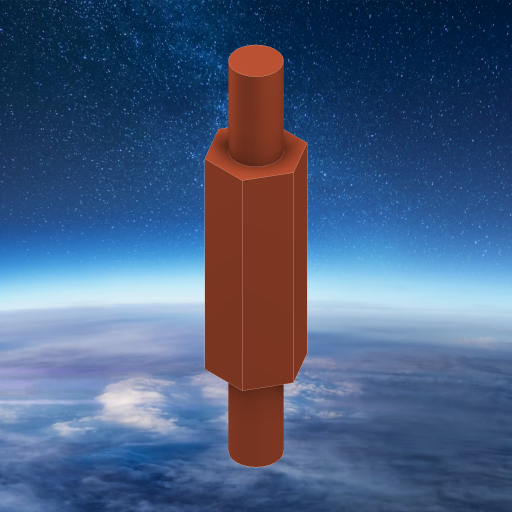
# Autodesk Inventor part: copper_pillar_M3_L15
Saved by Autodesk Inventor 2023 (Build 270158000, 158)
## iProperties
Created: 2022-11-08
Part Number: copper_pillar_M3_L15
Material: Copper
Document SubType Name: Modeling
Designer: 310611102
Density: 8.94 g/cm^3
Appearance: Copper - Satin
Mass: 3.46811 g
Surface Area: 3.98886 cm^2
Volume: 0.387932 cm^3
Author: 310611102
Autodesk Inventor part; units mm, degrees
ref_plane "YZ Plane" through (0, 0, 0) normal (1, 0, 0) x (0, 1, 0)
ref_plane "XZ Plane" through (0, 0, 0) normal (0, 1, 0) x (-1, 0, 0)
ref_plane "XY Plane" through (0, 0, 0) normal (0, 0, 1) x (1, 0, 0)
sketch "草圖2" plane through (0, 0, 0) normal (0, 1, 0) x (-1, 0, 0)
  line L0 (-2.8868, 0) -> (-1.4434, 2.5)
  line L1 (-1.4434, 2.5) -> (1.4434, 2.5)
  line L2 (1.4434, 2.5) -> (2.8868, 0)
  line L3 (2.8868, 0) -> (1.4434, -2.5)
  line L4 (1.4434, -2.5) -> (-1.4434, -2.5)
  line L5 (-1.4434, -2.5) -> (-2.8868, 0)
  point P0 (0, 0)
  point P1 (0, 0)
  dimension "d2" = 5
  constraints: 12 end point, 1 coincident, 13 other
  measures "d2" distance between parallel lines of L1 L4
extrude "擠出1" add sketch "草圖2" along normal blind 14
sketch "草圖3" plane through (0, 0, 0) normal (0, 0, 1) x (1, 0, 0)
  line L0 (1.4434, 14) -> (-1.4434, 14) projected
  line L1 (0, 14) -> (1.5, 14)
  line L2 (1.5, 14) -> (1.5, 20)
  line L3 (1.5, 20) -> (0, 20)
  line L4 (0, 20) -> (0, 14)
  line L5 (0, 17.268) -> (0, -3.3114)
  line L6 (0, 0) -> (1.5, 0)
  line L7 (1.5, 0) -> (1.5, -6)
  line L8 (1.5, -6) -> (0, -6)
  line L9 (0, -6) -> (0, 0)
  point P0 (0.75, 20)
  dimension "d5" = 3
  dimension "d6" = 6
  dimension "d8" = 6
  constraints: 18 end point, 4 parallel, 2 horizontal, 2 midpoint, 2 perpendicular, 1 collinear, 1 point on line, 1 vertical
  measures "d5" diameter of L2 L5
  measures "d6" distance from line of L0 point (0.75, 20)
  measures "d8" distance of L6.end L7.end
revolve "迴轉1" add sketch "草圖3" angle 360 about axis through (0, 17.268, 0) along (0, -1, 0)
